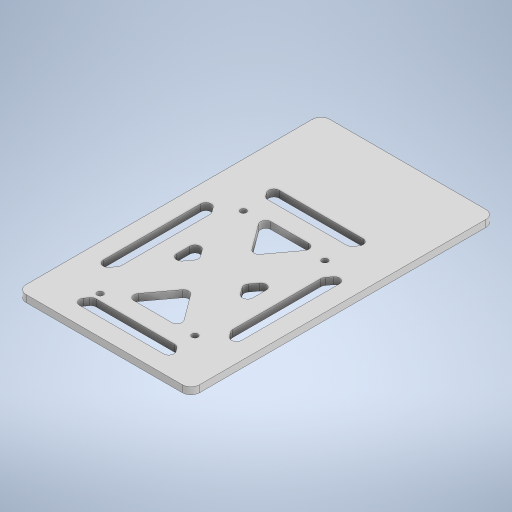
# Autodesk Inventor part: LI0014-ARDUINO SHELF
Saved by Autodesk Inventor 2023 (Build 270158000, 158)
## iProperties
Created: 2023-03-14
Part Number: LI0014-ARDUINO SHELF
Material: Generic
Document SubType Name: Modeling
Designer: Louis
Density: 1 g/cm^3
Appearance: Default
Author: Louis
Autodesk Inventor part; units mm, degrees
ref_plane "YZ Plane" through (0, 0, 0) normal (1, 0, 0) x (0, 1, 0)
ref_plane "XZ Plane" through (0, 0, 0) normal (0, 1, 0) x (-1, 0, 0)
ref_plane "XY Plane" through (0, 0, 0) normal (0, 0, 1) x (1, 0, 0)
sketch "Sketch1" plane through (0, 0, 0) normal (0, 1, 0) x (-1, 0, 0)
  line L0 (50, 67.5) -> (-50, 67.5)
  line L1 (-50, 67.5) -> (-50, -67.5)
  line L2 (-50, -67.5) -> (50, -67.5)
  line L3 (50, -67.5) -> (50, 67.5)
  point P0 (0, 0)
  point P1 (50, 0)
  point P2 (0, 67.5)
  dimension "d0" = 135
  dimension "d1" = 100
  constraints: 8 end point, 2 midpoint, 2 parallel, 1 horizontal, 1 horizontal alignment, 1 perpendicular, 1 vertical alignment
  measures "d0" distance of L2.end L0.start
  measures "d1" distance of L1.end L2.end
extrude "Extrusion1" add sketch "Sketch1" along normal blind 4
sketch "Sketch3" plane through (0, 4, 0) normal (0, 1, 0) x (1, 0, 0)
  line L0 (-26.67, 50.8) -> (26.67, 50.8)
  line L1 (26.67, 50.8) -> (26.67, -50.8)
  line L2 (26.67, -50.8) -> (-26.67, -50.8)
  line L3 (-26.67, -50.8) -> (-26.67, 50.8)
  point P0 (0, 0)
  point P1 (0, 50.8)
  point P2 (26.67, 0)
  point P3 (-24.13, 36.83)
  point P4 (24.147, 35.56)
  point P5 (24.147, -39.37)
  point P6 (-24.13, -45.72)
  dimension "d11" = 53.34
  dimension "d40" = 13.97
  dimension "d42" = 101.6
  dimension "d48" = 2.54
  dimension "d49" = 15.24
  dimension "d50" = 2.523
  dimension "d56" = 90.17
  dimension "d57" = 96.52
  constraints: 8 end point, 3 vertical alignment, 2 midpoint, 2 parallel, 1 horizontal, 1 horizontal alignment, 1 perpendicular
  measures "d11" distance of L0.start L0.end
  measures "d40" distance from line of L0 point (-24.13, 36.83)
  measures "d42" distance of L0.end L1.end
  measures "d48" distance from line of L3 point (-24.13, 36.83)
  measures "d49" distance from line of L0 point (24.147, 35.56)
  measures "d50" distance from line of L1 point (24.147, 35.56)
  measures "d56" distance from line of L0 point (24.147, -39.37)
  measures "d57" distance from line of L0 point (-24.13, -45.72)
hole "Hole1" at (-24.13, 4, -36.83) at (24.147, 4, -35.56) at (24.147, 4, 39.37) at (-24.13, 4, 45.72) direction (0, -1, 0) diameter 3.4 end through all clearance for "Flat Head Machine Screw" size "M3" standard "Ansi Metric M Profile"
sketch "Sketch4" plane through (0, 4, 0) normal (0, 1, 0) x (1, 0, 0)
  line L0 (-32, 49.5) -> (32, 49.5)
  line L1 (32, 49.5) -> (32, -49.5)
  line L2 (32, -49.5) -> (-32, -49.5)
  line L3 (-32, -49.5) -> (-32, 49.5)
  line L4 (-50, 67.5) -> (50, 67.5)
  line L5 (50, 67.5) -> (50, -67.5)
  line L6 (50, -67.5) -> (-50, -67.5)
  line L7 (-50, -67.5) -> (-50, 67.5)
  line L8 (50, -67.5) -> (50, 67.5) projected
  line L9 (50, 67.5) -> (-50, 67.5) projected
  line L10 (-50, 67.5) -> (-50, -67.5) projected
  line L11 (-50, -67.5) -> (50, -67.5) projected
  line L12 (40, 57.5) -> (-40, 57.5)
  line L13 (-40, 57.5) -> (-40, -57.5)
  line L14 (-40, -57.5) -> (40, -57.5)
  line L15 (40, -57.5) -> (40, 57.5)
  line L16 (22, 39.5) -> (-22, 39.5)
  line L17 (-22, 39.5) -> (-22, -39.5)
  line L18 (-22, -39.5) -> (22, -39.5)
  line L19 (22, -39.5) -> (22, 39.5)
  line L20 (-50, 67.5) -> (50, -67.5)
  line L21 (50, 67.5) -> (-50, -67.5)
  line L22 (41.9644, 73.4523) -> (-58.0356, -61.5477)
  line L23 (58.0356, 61.5477) -> (-41.9644, -73.4523)
  line L24 (-41.9644, 73.4523) -> (58.0356, -61.5477)
  line L25 (-58.0356, 61.5477) -> (41.9644, -73.4523)
  point P0 (0, 0)
  point P1 (0, 49.5)
  point P2 (32, 0)
  point P3 (50, -62.5)
  point P4 (50, 62.5)
  point P5 (45, 67.5)
  point P6 (-45, 67.5)
  point P7 (-50, 62.5)
  point P8 (-50, -62.5)
  point P9 (-45, -67.5)
  point P10 (45, -67.5)
  point P11 (21.67, -37.6546)
  point P12 (0, -16.8003)
  point P13 (-21.67, -37.6546)
  point P14 (-12.4447, 0)
  point P15 (-22, 12.8997)
  point P16 (-22, -12.8997)
  point P17 (-21.67, 37.6546)
  point P18 (0, 16.8003)
  point P19 (21.67, 37.6546)
  point P20 (12.4447, 0)
  point P21 (22, -12.8997)
  point P22 (22, 12.8997)
  point P23 (40, -37.1997)
  point P24 (40, 37.1997)
  point P25 (30.1479, -57.5)
  point P26 (-30.1479, -57.5)
  point P27 (-40, 37.1997)
  point P28 (-40, -37.1997)
  point P29 (-30.1479, 57.5)
  point P30 (30.1479, 57.5)
  point P31 (-16.8146, 39.5)
  point P32 (16.8146, 39.5)
  point P33 (16.8146, -39.5)
  point P34 (-16.8146, -39.5)
  point P35 (24.222, -49.5)
  point P36 (-24.222, -49.5)
  point P37 (-24.222, 49.5)
  point P38 (24.222, 49.5)
  point P39 (-32, 26.3997)
  point P40 (-32, -26.3997)
  point P41 (32, -26.3997)
  point P42 (32, 26.3997)
  dimension "d27" = 10
  dimension "d29" = 10
  dimension "d30" = 10
  dimension "d31" = 10
  dimension "d32" = 10
  dimension "d33" = 10
  dimension "d58" = 8
  dimension "d59" = 8
  constraints: 44 end point, 12 parallel, 4 collinear, 4 perpendicular, 2 horizontal, 2 midpoint, 1 horizontal alignment, 1 vertical alignment, 6 other
  measures "d27" distance between parallel lines of L4 L12
  measures "d29" distance between parallel lines of L0 L16
  measures "d30" distance between parallel lines of L21 L22
  measures "d31" distance between parallel lines of L21 L23
  measures "d32" distance between parallel lines of L20 L24
  measures "d33" distance between parallel lines of L20 L25
  measures "d58" distance between parallel lines of L13 L3
  measures "d59" distance between parallel lines of L12 L0
extrude "Extrusion3" cut sketch "Sketch4" against normal through all contours L24 L12 L22 L0 | L16 L22 L24 | L3 L22 L13 L25 | L25 L22 L17 | L23 L15 L24 L1 | L23 L19 L24 | L2 L25 L14 L23 | L25 L18 L23
thicken "Thicken1" operation add thickness 40 both sides no extend neighbours no toward (0, 0, -1) faces at (16.6667, 1.3333, -67.5)
fillet "Fillet4" radius 5 4 edges at (50, 2, 67.5) (50, 2, -107.5) (-50, 2, -107.5) (-50, 2, 67.5)
fillet "Fillet5" radius 3 28 edges at (-22, 2, 12.8997) (-22, 2, -12.8997) (-12.4447, 2, 0) (16.8146, 2, -39.5) (22, 2, -12.8997) (12.4447, 2, 0) (22, 2, 12.8997) (0, 2, -16.8003) (-16.8146, 2, -39.5) (-40, 2, -37.1997) (-32, 2, -26.3997) (-32, 2, 26.3997) (-40, 2, 37.1997) (-16.8146, 2, 39.5) (0, 2, 16.8003) (24.222, 2, 49.5) (32, 2, -26.3997) (16.8146, 2, 39.5) (30.1479, 2, 57.5) (-30.1479, 2, 57.5) (-24.222, 2, 49.5) (40, 2, -37.1997) (40, 2, 37.1997) (32, 2, 26.3997) (24.222, 2, -49.5) (30.1479, 2, -57.5) (-30.1479, 2, -57.5) (-24.222, 2, -49.5)
body "Solid1"
